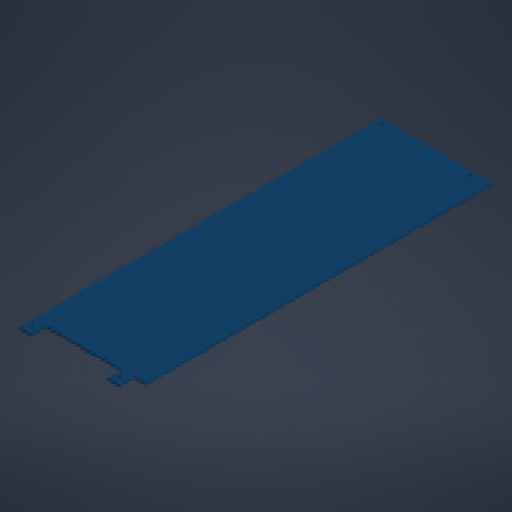
# Autodesk Inventor part: pcb
Saved by Autodesk Inventor 2026.2 (Build 302298000, 298)
## iProperties
Created: 2025-12-21
Part Number: pcb
Material: Ogólny
Document SubType Name: Modeling
Designer: test
Density: 1 g/cm^3
Appearance: Domyślna
Author: test
Autodesk Inventor part; units mm, degrees
ref_plane "YZ Plane" through (0, 0, 0) normal (1, 0, 0) x (0, 1, 0)
ref_plane "XZ Plane" through (0, 0, 0) normal (0, 1, 0) x (-1, 0, 0)
ref_plane "XY Plane" through (0, 0, 0) normal (0, 0, 1) x (1, 0, 0)
sketch "Szkic1" plane through (0, 0, 0) normal (0, 1, 0) x (-1, 0, 0)
  line L0 (0, 0) -> (85.11, 0)
  line L1 (85.11, 0) -> (85.11, 274.11)
  line L2 (85.11, 274.11) -> (75.98, 274.11)
  line L3 (75.98, 274.11) -> (75.98, 263.11)
  line L4 (75.98, 263.11) -> (18.11, 263.11)
  line L5 (18.11, 263.11) -> (18.11, 274.11)
  line L6 (18.11, 274.11) -> (8.98, 274.11)
  line L7 (8.98, 274.11) -> (8.98, 263.11)
  line L8 (8.98, 263.11) -> (0, 263.11)
  line L9 (0, 263.11) -> (0, 0)
  point P0 (80.545, 274.11)
  point P1 (13.545, 274.11)
  dimension "d0" = 274.11
  dimension "d1" = 85.11
  dimension "d2" = 11
  dimension "d3" = 9.13
  dimension "d4" = 9.13
  dimension "d5" = 67
  constraints: 20 end point, 7 perpendicular, 3 point on line, 2 midpoint, 1 horizontal, 1 parallel
  measures "d0" distance between parallel lines of L0 L2
  measures "d1" distance between parallel lines of L1 L9
  measures "d2" distance between parallel lines of L2 L4
  measures "d3" distance between parallel lines of L1 L3
  measures "d4" distance between parallel lines of L7 L5
  measures "d5" distance of point (80.545, 274.11) point (13.545, 274.11)
extrude "Wyciągnięcie proste1" add sketch "Szkic1" along normal blind 1.7
sketch "Sketch2" plane through (0, 1.7, 0) normal (0, 1, 0) x (1, 0, 0)
  line L0 (-80.545, -269.61) -> (-13.545, -269.61) construction
  line L1 (-13.545, -269.61) -> (-13.545, -4.5) construction
  line L2 (-13.545, -4.5) -> (-80.545, -4.5) construction
  line L3 (-80.545, -4.5) -> (-80.545, -269.61) construction
  line L4 (-85.11, -274.11) -> (-75.98, -274.11) projected
  line L5 (0, 0) -> (-85.11, 0) projected
  line L6 (-75.98, -274.11) -> (-75.98, -263.11) projected
  line L7 (-85.11, 0) -> (-85.11, -274.11) projected
  line L8 (-8.98, -274.11) -> (-8.98, -263.11) projected
  dimension "d15" = 4.5
  dimension "d16" = 4.5
  dimension "d18" = 9.13
  dimension "d19" = 4.565
  dimension "d20" = 4.565
  constraints: 8 end point, 2 coincident, 2 parallel, 1 horizontal, 1 perpendicular
  measures "d15" distance between parallel lines of L4 L0
  measures "d16" distance between parallel lines of L2 L5
  measures "d18" distance between parallel lines of L6 L7
  measures "d19" distance between parallel lines of L7 L3
  measures "d20" distance between parallel lines of L8 L1
hole "Hole1" at (-80.545, 1.7, 269.61) at (-13.545, 1.7, 269.61) at (-13.545, 1.7, 4.5) at (-80.545, 1.7, 4.5) direction (0, -1, 0) diameter 3.5 depth 1.7
equation "\"d4\" = d3"
equation "\"d19\" = 0.5 * d18"
equation "\"d20\" = d19"
